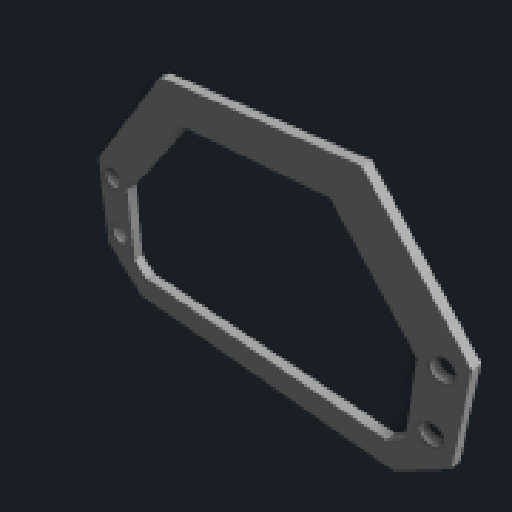
# Autodesk Inventor part: JawMount
Saved by Autodesk Inventor 2025.2 (Build 292293000, 293)
## iProperties
Created: 2024-12-21
Part Number: JawMount
Material: Generic
Document SubType Name: Sheet Metal
Designer: valer
Density: 1 g/cm^3
Sheet Metal Rule: Default
Appearance: Default
Author: valer
Autodesk Inventor part; units mm, degrees
ref_plane "YZ Plane" through (0, 0, 0) normal (1, 0, 0) x (0, 1, 0)
ref_plane "XZ Plane" through (0, 0, 0) normal (0, 1, 0) x (-1, 0, 0)
ref_plane "XY Plane" through (0, 0, 0) normal (0, 0, 1) x (1, 0, 0)
sketch "Sketch1" plane through (0, 0, 0) normal (0, 0, 1) x (1, 0, 0)
  circle A0 centre (-3.2439, -112.6362) radius 2.7 construction
  circle A1 centre (-3.2439, -130.6362) radius 2.7 construction
  line L0 (-22.4336, -106.6362) -> (-3.2439, -106.6362) construction
  line L1 (-3.2439, -136.6362) -> (-18.3318, -136.6362) construction
  line L2 (49.7615, -342.4426) -> (49.7615, 314.6303) construction
  line L3 (-9.2439, -108.8185) -> (-9.2439, -136.6362)
  line L4 (-9.2439, -136.6362) -> (2.7561, -136.6362) construction
  line L5 (2.7561, -136.6362) -> (2.7561, -113.501)
  line L6 (-9.2439, -108.8185) -> (20.3828, -76.6362)
  line L7 (20.3828, -76.6362) -> (49.7615, -76.6362)
  line L8 (2.7561, -113.501) -> (27.4876, -86.6362)
  line L9 (27.4876, -86.6362) -> (49.7615, -86.6362)
  line L10 (14.6694, -102.2191) -> (33.1572, -82.1367) construction
  line L11 (2.7561, -112.6362) -> (2.7561, -130.6362) construction
  circle A2 centre (-3.2439, -112.6362) radius 3
  circle A3 centre (-3.2439, -130.6362) radius 3
  line L12 (2.7561, -136.6362) -> (6.2838, -140.6362)
  line L13 (6.2838, -140.6362) -> (49.7615, -140.6362)
  line L14 (-9.2439, -136.6362) -> (1.3391, -148.6362)
  line L15 (1.3391, -148.6362) -> (49.7615, -148.6362)
  line L16 (108.7669, -108.8185) -> (108.7669, -136.6362)
  line L17 (96.7669, -136.6362) -> (96.7669, -113.501)
  line L18 (108.7669, -108.8185) -> (79.1402, -76.6362)
  line L19 (79.1402, -76.6362) -> (49.7615, -76.6362)
  line L20 (96.7669, -113.501) -> (72.0355, -86.6362)
  line L21 (72.0355, -86.6362) -> (49.7615, -86.6362)
  circle A4 centre (102.7669, -112.6362) radius 3
  circle A5 centre (102.7669, -130.6362) radius 3
  line L22 (96.7669, -136.6362) -> (93.2393, -140.6362)
  line L23 (93.2393, -140.6362) -> (49.7615, -140.6362)
  line L24 (108.7669, -136.6362) -> (98.1839, -148.6362)
  line L25 (98.1839, -148.6362) -> (49.7615, -148.6362)
  line L26 (27.4876, -86.6362) -> (49.7615, -140.6362)
  line L27 (18.5234, -96.3737) -> (36.7808, -140.6362)
  line L28 (72.0355, -86.6362) -> (49.7615, -140.6362)
  line L29 (80.9997, -96.3737) -> (62.7423, -140.6362)
  point P0 (0, 0)
  point P1 (-12.8387, -106.6362)
  dimension "d0" = 6
  dimension "d1" = 6
  dimension "d2" = 9
  dimension "d3" = 8
  dimension "d4" = 4
  dimension "d5" = 10
  dimension "d6" = 12
  dimension "d7" = 12
  dimension "d8" = 7
  dimension "d9" = 20
  dimension "d11" = 12
  measures "d0" diameter of A2
  measures "d1" diameter of A3
  measures "d2" distance between parallel lines of L14 L12
  measures "d3" distance between parallel lines of L15 L13
  measures "d4" distance between parallel lines of L13 L4
  measures "d5" distance between parallel lines of L7 L9
  measures "d6" distance between parallel lines of L6 L8
  measures "d7" distance between parallel lines of L3 L11
  measures "d8" distance from line of L6 A0.centre
  measures "d9" distance from line of L9 point (-12.839, -106.636)
  measures "d11" distance between parallel lines of L27 L26
extrude "Plate1" add sketch "Sketch1" along normal blind 3.048 contours L6 L7 L19 L18 L16 L24 L25 L15 L14 L3 | L8 L26 L13 L27 | L28 L20 L29 L23
chamfer "Chamfer1" distance 4 angle 45 9 edges at (18.5234, -96.3737, 1.524) (72.0355, -86.6362, 1.524) (27.4876, -86.6362, 1.524) (80.9997, -96.3737, 1.524) (62.7423, -140.6362, 1.524) (36.7808, -140.6362, 1.524) (49.7615, -140.6362, 1.524) (20.3828, -76.6362, 1.524) (79.1402, -76.6362, 1.524)
fillet "Fillet1" radius 4 30 edges at (-9.2439, -136.6362, 1.524) (-9.2439, -108.8185, 1.524) (17.6737, -79.5791, 1.524) (24.3828, -76.6362, 1.524) (75.1402, -76.6362, 1.524) (81.8494, -79.5791, 1.524) (108.7669, -108.8185, 1.524) (108.7669, -136.6362, 1.524) (98.1839, -148.6362, 1.524) (1.3391, -148.6362, 1.524) (51.2868, -136.9384, 1.524) (48.2363, -136.9384, 1.524) (70.5102, -90.334, 1.524) (68.0355, -86.6362, 1.524) (31.4876, -86.6362, 1.524) (29.0129, -90.334, 1.524) (79.4744, -100.0715, 1.524) (64.2676, -136.9384, 1.524) (83.7089, -99.3166, 1.524) (96.7669, -113.501, 1.524) (96.7669, -136.6362, 1.524) (93.2393, -140.6362, 1.524) (66.7423, -140.6362, 1.524) (6.2838, -140.6362, 1.524) (2.7561, -136.6362, 1.524) (2.7561, -113.501, 1.524) (32.7808, -140.6362, 1.524) (35.2555, -136.9384, 1.524) (20.0486, -100.0715, 1.524) (15.8142, -99.3166, 1.524)
equation "\"d10\" = Thickness"
equation "\"BendRadius\" = Thickness"
equation "\"BendReliefWidth\" = Thickness"
equation "\"BendReliefDepth\" = 0.5 * Thickness"
equation "\"CornerReliefSize\" = 4 * Thickness"
equation "\"MinimumRemnant\" = 2 * Thickness"
equation "\"TransitionRadius\" = BendRadius"
equation "\"JacobiRadiusSize\" = BendRadius"
equation "\"GapSize\" = Thickness"
equation "\"Thickness\" = 3.048"
body "Solid1"
